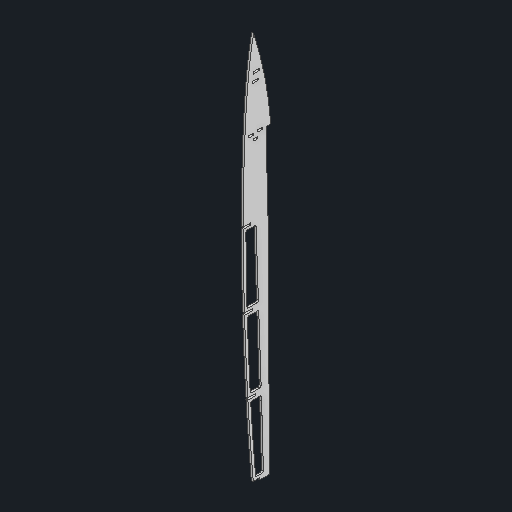
# Autodesk Inventor part: stringer
Saved by Autodesk Inventor 2024 (Build 280153000, 153)
## iProperties
Created: 2022-03-21
Part Number: stringer
Material: Generic
Document SubType Name: Modeling
Designer: kardo
Density: 1 g/cm^3
Appearance: Default
Mass: 41.3524 g
Surface Area: 339.584 cm^2
Volume: 41.3524 cm^3
Author: kardo
Autodesk Inventor part; units mm, degrees
ref_plane "YZ Plane" through (0, 0, 0) normal (1, 0, 0) x (0, 1, 0)
ref_plane "XZ Plane" through (0, 0, 0) normal (0, 1, 0) x (-1, 0, 0)
ref_plane "XY Plane" through (0, 0, 0) normal (0, 0, 1) x (1, 0, 0)
derived "parameters_frame.ipt"
derived "surface_body.ipt"
sketch "sk_long_outer" plane through (0, 0, 0) normal (1, 0, 0) x (0, 1, 0)
  line L0 (-345, 107.6209) -> (-345, -224.5198) construction
  line L1 (255, 107.6209) -> (255, -224.5198) construction
  line L2 (-465, 54.4) -> (375, 54.4) construction
  line L3 (-483, 0) -> (357, 0) construction
  line L4 (0, 107.6209) -> (0, -224.5198) construction
  line L5 (0, 14.144) -> (-345, 11.968)
  line L6 (-345, 11.968) -> (-345, 39.712)
  line L7 (-345, 39.712) -> (0, 54.4)
  line L8 (0, 54.4) -> (255, 36.448)
  line L9 (0, 0) -> (122.4, 9.6331)
  line L10 (122.4, 9.6331) -> (255, 36.448)
  line L11 (0, 14.144) -> (0, 0)
  line L12 (0, 14.144) -> (121.9006, 15.9783)
  line L13 (121.9006, 15.9783) -> (122.4, 9.6331)
sketch "sk_rail_sponson_tunnel" plane through (81.12, 0, 0) normal (1, 0, 0) x (0, 1, 0)
  line L0 (0, 0) -> (122.4, 9.6331)
  line L1 (111.1171, 152.996) -> (142.2856, -243.0375) construction
  spline S0 degree 2 poles (122.4, 9.6331) (190.08, 14.9596) (255, 36.448) knots 0 0 0 1 1 1
sketch "sk_rail_top_tunnel" plane through (81.12, 0, 0) normal (1, 0, 0) x (0, 1, 0)
  line L0 (255, 107.6209) -> (255, -224.5198) construction
  line L1 (0, 107.6209) -> (0, -224.5198) construction
  line L2 (-345, 107.6209) -> (-345, -224.5198) construction
  line L3 (-345, 0) -> (0, 0) construction
  line L4 (-172.5, 48.8998) -> (-172.5, 0) construction
  line L5 (0, 52.89) -> (37.026, 52.89) construction
  line L6 (37.026, 52.89) -> (80.784, 47.0555) construction
  line L7 (80.784, 47.0555) -> (112.2, 37.536) construction
  line L8 (112.2, 107.6209) -> (112.2, -224.5198) construction
  line L9 (0, 52.89) -> (255, 52.89) construction
  line L10 (-469.9275, 0) -> (379.2584, 0) construction
  spline S0 degree 3 poles (0, 52.89) (92.8353, 52.89) (195.0311, 49.5089) (255, 36.448) knots 0 0 0 0 1 1 1 1
  spline S1 degree 3 poles (0, 52.89) (37.026, 52.89) (80.784, 47.0555) (112.2, 37.536) knots 1 1 1 1 2 2 2 2
  spline S2 degree 4 poles (-345, 37.3935) (-258.8686, 45.1235) (-172.5923, 49.7074) (-86.3167, 52.89) (0, 52.89) knots 0 0 0 0 0 1 1 1 1 1
  point P0 (153, 48.7795)
  point P1 (112.2, 28.832)
  point P2 (-230.0001, 45.8224)
  point P3 (-114.9999, 50.9907)
sketch "sk_rail_bottom_tunnel" plane through (81.12, 0, 0) normal (1, 0, 0) x (0, 1, 0)
  line L0 (-241.5001, 19.2432) -> (11.22, 28.376)
  arc A0 (36.465, 28.832) -> (11.22, 28.376) centre (36.465, -670.197) ccw
  line L1 (36.465, 28.832) -> (112.2, 28.832)
  arc A1 (-262.2001, 18.586) -> (-241.5001, 19.2432) centre (-326.8578, 2381.2399) ccw
  line L2 (-345, 16.32) -> (-262.2001, 18.586)
  point P0 (0, 0)
ref_plane "plane_middle" through (0, 0, 0) normal (0, 1, 0) x (-1, 0, 0)
ref_plane "plane_tunnel_right" through (81.12, 0, 0) normal (1, 0, 0) x (0, 1, 0)
ref_plane "plane_tail_1" through (0, -114.9999, 0) normal (0, 1, 0) x (-1, 0, 0)
ref_plane "plane_tail_2" through (0, -230.0001, 0) normal (0, 1, 0) x (-1, 0, 0)
derived "stencil_frame.ipt"
sketch "sk_joint_locations" plane through (81.12, 0, 0) normal (1, 0, 0) x (0, 1, 0)
  line L0 (0, 0) -> (122.4, 9.6331) construction
  line L1 (36.465, 28.832) -> (112.2, 28.832) construction
  arc A0 (36.465, 28.832) -> (11.22, 28.376) centre (36.465, -670.197) ccw construction
  line L2 (-241.5001, 19.2432) -> (11.22, 28.376) construction
  line L3 (-345, 16.32) -> (-262.2001, 18.586) construction
  arc A1 (-262.2001, 18.586) -> (-241.5001, 19.2432) centre (-326.8578, 2381.2399) ccw construction
  line L4 (-122.4795, 3121.122) -> (270.8781, -1876.9598) construction
  line L5 (-230.0001, 3089.1136) -> (-230.0001, -1866.0023) construction
  line L6 (-114.9999, 3089.1136) -> (-114.9999, -1866.0023) construction
  line L7 (-345, 3089.1136) -> (-345, -1866.0023) construction
  line L8 (0, 3089.1136) -> (0, -1866.0023) construction
  line L9 (529.622, 47.2379) -> (-602.608, 2.7525) construction
  line L10 (-673.1615, -36.5999) -> (647.9226, 67.3717) construction
  line L11 (189.4528, 29.5173) -> (189.1111, 38.2146) construction
  line L12 (201.105, 36.5853) -> (201.7901, 27.8813) construction
  line L13 (0, 14.144) -> (121.9006, 15.9783) construction
  line L14 (-230.0001, 45.8224) -> (-230.0001, 19.6588) construction
  line L15 (-345, 37.3935) -> (-345, 16.32) construction
  line L16 (-114.9999, 50.9907) -> (-114.9999, 23.8147) construction
  line L17 (0, 52.89) -> (0, 27.9705) construction
  line L18 (119.1768, 50.5875) -> (119.7216, 43.6656) construction
  line L19 (120.2663, 36.7438) -> (119.7216, 43.6656) construction
  line L20 (120.2663, 36.7438) -> (120.8111, 29.822) construction
  line L21 (120.8111, 29.822) -> (121.3559, 22.9001) construction
  line L22 (121.3559, 22.9001) -> (121.9006, 15.9783) construction
  line L23 (0, 14.144) -> (0, 0) construction
  spline S0 degree 4 poles (-345, 37.3935) (-258.8686, 45.1235) (-172.5923, 49.7074) (-86.3167, 52.89) (0, 52.89) knots 0 0 0 0 0 1 1 1 1 1
  spline S1 degree 3 poles (0, 52.89) (92.8353, 52.89) (195.0311, 49.5089) (255, 36.448) knots 0 0 0 0 1 1 1 1
  spline S2 degree 2 poles (122.4, 9.6331) (190.08, 14.9596) (255, 36.448) knots 0 0 0 1 1 1
  line L24 (112.2, 37.536) -> (112.2, 28.832) construction
  line L25 (112.2, 35.848) -> (112.2, 30.52) construction
  point P0 (189.282, 33.8659)
  point P1 (201.4475, 32.2333)
  point P2 (-345, 26.8568)
  point P3 (-230.0001, 32.7406)
  point P4 (-114.9999, 37.4027)
  point P5 (0, 40.4303)
  point P6 (112.2, 33.184)
sketch "sk_stringer_base" plane through (81.12, 0, 0) normal (1, 0, 0) x (0, 1, 0)
  line L0 (0, 14.144) -> (-345, 11.968) construction
  spline S0 degree 4 poles (-345, 37.3935) (-258.8686, 45.1235) (-172.5923, 49.7074) (-86.3167, 52.89) (0, 52.89) knots 0 0 0 0 0 1 1 1 1 1 construction
  spline S1 degree 3 poles (0, 52.89) (37.026, 52.89) (80.784, 47.0555) (112.2, 37.536) knots 1 1 1 1 2 2 2 2 construction
  spline S2 degree 3 poles (0, 52.89) (92.8353, 52.89) (195.0311, 49.5089) (255, 36.448) knots 0 0 0 0 1 1 1 1 construction
  spline S3 degree 2 poles (122.4, 9.6331) (190.08, 14.9596) (255, 36.448) knots 0 0 0 1 1 1 construction
  line L1 (0, 0) -> (122.4, 9.6331) construction
  line L2 (-345, 16.32) -> (-262.2001, 18.586) construction
  arc A0 (-262.2001, 18.586) -> (-241.5001, 19.2432) centre (-326.8578, 2381.2399) ccw construction
  line L3 (-241.5001, 19.2432) -> (11.22, 28.376) construction
  arc A1 (36.465, 28.832) -> (11.22, 28.376) centre (36.465, -670.197) ccw construction
  line L4 (36.465, 28.832) -> (112.2, 28.832) construction
  line L5 (0, 2991.5273) -> (0, -1280.4843) construction
  line L6 (-345, 26.8568) -> (-345, 11.968)
  line L7 (-345, 11.968) -> (0, 14.144)
  line L8 (119.3465, 10.1952) -> (118.832, 16.7322)
  line L9 (0, 14.144) -> (0, 14.944)
  line L10 (0, 14.944) -> (118.832, 16.7322)
  line L11 (-345, 26.8568) -> (-342, 26.8568)
  line L12 (-342, 26.8568) -> (-342, 36.8582)
  line L13 (-230.0001, 32.7406) -> (-227.0001, 32.7406)
  line L14 (-227.0001, 32.7406) -> (-227.0001, 45.1951)
  line L15 (-230.0001, 32.7406) -> (-230.0001, 45.0211)
  line L16 (-114.9999, 37.4027) -> (-114.9999, 50.1903)
  line L17 (-114.9999, 37.4027) -> (-111.9999, 37.4027)
  line L18 (-111.9999, 37.4027) -> (-111.9999, 50.2837)
  line L19 (0, 52.09) -> (0, 40.4303)
  line L20 (0, 40.4303) -> (3, 40.4303)
  line L21 (3, 40.4303) -> (3, 52.0888)
  line L22 (119.7216, 43.6656) -> (120.2663, 36.7438)
  line L23 (120.2663, 36.7438) -> (117.2756, 36.5084)
  line L24 (117.2756, 36.5084) -> (116.7308, 43.4303)
  line L25 (116.7308, 43.4303) -> (119.7216, 43.6656)
  line L26 (120.8111, 29.822) -> (117.8203, 29.5866)
  line L27 (117.8203, 29.5866) -> (118.3651, 22.6647)
  line L28 (118.3651, 22.6647) -> (121.3559, 22.9001)
  line L29 (120.8111, 29.822) -> (121.3559, 22.9001)
  line L30 (189.1111, 38.2146) -> (189.4528, 29.5173)
  line L31 (201.105, 36.5853) -> (201.7901, 27.8813)
  line L32 (201.7901, 27.8813) -> (198.7993, 27.646)
  line L33 (198.7993, 27.646) -> (198.1143, 36.35)
  line L34 (198.1143, 36.35) -> (201.105, 36.5853)
  line L35 (189.1111, 38.2146) -> (186.1134, 38.0968)
  line L36 (186.1134, 38.0968) -> (186.4551, 29.3995)
  line L37 (186.4551, 29.3995) -> (189.4528, 29.5173)
  line L38 (122.3372, 10.4306) -> (119.3465, 10.1952)
  line L39 (109.2, 35.848) -> (112.2, 35.848)
  line L40 (112.2, 35.848) -> (112.2, 30.52)
  line L41 (112.2, 30.52) -> (109.2, 30.52)
  line L42 (109.2, 30.52) -> (109.2, 35.848)
  spline S4 degree 5 poles (-342, 36.8582) (-273.7802, 42.9173) (-205.3987, 47.149) (-136.9758, 50.2102) (-68.4884, 52.0902) (0, 52.09) knots 0 0 0 0 0 0 1 1 1 1 1 1
  spline S5 degree 5 poles (0, 52.09) (14.1126, 52.09) (28.2252, 52.0249) (42.3374, 51.8877) (70.3021, 51.4557) (98.2587, 50.655) (112.105, 50.1551) (138.5853, 48.9703) (165.0353, 47.2425) (177.6496, 46.2711) (200.7384, 44.1675) (223.7378, 41.2476) (234.1569, 39.7078) (244.5404, 37.9065) (254.8298, 35.6663) knots 0 0 0 0 0 0 0.275917 0.275917 0.275917 0.546795 0.546795 0.546795 0.794123 0.794123 0.794123 1 1 1 1 1 1
  spline S6 degree 4 poles (254.7486, 37.2075) (222.6091, 26.5695) (189.6306, 18.4466) (156.0872, 13.0866) (122.3372, 10.4306) knots 0 0 0 0 0 1 1 1 1 1
  point P0 (251.9318, 36.2831)
  point P1 (121.9006, 15.9783)
  dimension "d4" = 0.8
  dimension "d14" = 0.8
  dimension "d8" = 0.8
  dimension "d9" = 3
  dimension "d11" = 3
  dimension "d16" = 3
  dimension "d17" = 0.8
  constraints: 74 end point, 12 perpendicular, 7 vertical, 6 equal length, 6 parallel, 2 coincident, 2 collinear, 2 horizontal, 18 other
  measures "d8" distance of L7.end L9.end
  measures "d9" distance of L6.start L11.end
  measures "d11" distance of L19.end L20.end
  measures "d16" distance between parallel lines of L40 L42
  measures "d17" distance from line of point (121.901, 15.978) L10
extrude "thicken" add sketch "sk_stringer_base" along normal blind 3 contours L11 L12 S4 L15 L13 L14 L16 L17 L18 L19 L20 L21 S5 S6 L38 L8 L10 L9 L7 L6
sketch "sk_cut_weight" plane through (81.12, 0, 0) normal (1, 0, 0) x (0, 1, 0)
  spline S0 degree 4 poles (-345, 37.3935) (-258.8686, 45.1235) (-172.5923, 49.7074) (-86.3167, 52.89) (0, 52.89) knots 0 0 0 0 0 1 1 1 1 1 construction
  spline S1 degree 3 poles (0, 52.89) (37.026, 52.89) (80.784, 47.0555) (112.2, 37.536) knots 1 1 1 1 2 2 2 2 construction
  line L0 (36.465, 28.832) -> (112.2, 28.832) construction
  arc A0 (36.465, 28.832) -> (11.22, 28.376) centre (36.465, -670.197) ccw construction
  line L1 (-241.5001, 19.2432) -> (11.22, 28.376) construction
  arc A1 (-262.2001, 18.586) -> (-241.5001, 19.2432) centre (-326.8578, 2381.2399) ccw construction
  line L2 (-345, 16.32) -> (-262.2001, 18.586) construction
  line L3 (112.2, 37.536) -> (112.2, 28.832) construction
  line L4 (108.4873, 33.632) -> (36.465, 33.632)
  arc A2 (36.465, 33.632) -> (11.0467, 33.1729) centre (36.465, -670.197) ccw
  line L5 (11.0467, 33.1729) -> (-241.6735, 24.0401)
  arc A3 (-262.3314, 23.3842) -> (-241.6735, 24.0401) centre (-326.8578, 2381.2399) ccw
  line L6 (-262.3314, 23.3842) -> (-338, 21.3134)
  line L7 (-345, 16.32) -> (-345, 37.3935) construction
  line L8 (-342, 46.2922) -> (-342, 7.6751) construction
  line L9 (-227.0001, 59.5201) -> (-227.0001, 2.898) construction
  line L10 (-111.9999, 68.9991) -> (-111.9999, 15.2181) construction
  line L11 (0, 2991.5273) -> (0, -1280.4843) construction
  line L12 (-230.0001, 2991.5273) -> (-230.0001, -1280.4843) construction
  line L13 (-114.9999, 2991.5273) -> (-114.9999, -1280.4843) construction
  line L14 (-338, 21.3134) -> (-338, 33.1956)
  line L15 (-234.0001, 40.7786) -> (-234.0001, 24.3174)
  line L16 (-223.0001, 41.4174) -> (-223.0001, 24.7149)
  line L17 (-118.9999, 46.0602) -> (-118.9999, 28.4733)
  line L18 (-107.9999, 46.4032) -> (-107.9999, 28.8708)
  line L19 (-4, 48.0874) -> (-4, 32.6291)
  spline S2 degree 5 poles (-338, 33.1956) (-270.5733, 39.1068) (-202.9921, 43.2515) (-135.37, 46.2518) (-67.6854, 48.0902) (0, 48.09) knots 0 0 0 0 0 0 1 1 1 1 1 1
  spline S3 degree 5 poles (0, 48.09) (7.6357, 48.0899) (15.2714, 47.8806) (22.8997, 47.4965) (38.2518, 46.3949) (53.5443, 44.6516) (61.2292, 43.6141) (75.3782, 41.394) (89.4128, 38.543) (95.8175, 37.089) (102.1841, 35.4696) (108.4873, 33.632) knots 0 0 0 0 0 0 0.347809 0.347809 0.347809 0.700936 0.700936 0.700936 1 1 1 1 1 1
  point P0 (0, 0)
  dimension "d20" = 4.8
  dimension "d21" = 3
  dimension "d22" = 3
  dimension "d23" = 3
  dimension "d25" = 4
  dimension "d26" = 4
  dimension "d27" = 4
  dimension "d28" = 4
  dimension "d29" = 4
  dimension "d30" = 4
  constraints: 29 end point, 10 parallel, 5 point on line, 4 point on circle, 2 centre point, 16 other
  measures "d21" distance between parallel lines of L7 L8
  measures "d22" distance between parallel lines of L12 L9
  measures "d23" distance between parallel lines of L13 L10
  measures "d25" distance between parallel lines of L8 L14
  measures "d26" distance between parallel lines of L12 L15
  measures "d27" distance between parallel lines of L9 L16
  measures "d28" distance between parallel lines of L17 L13
  measures "d29" distance between parallel lines of L18 L10
  measures "d30" distance between parallel lines of L19 L11
extrude "cut_weight" cut sketch "sk_cut_weight" along normal through all both and the other way through all contours L19 L5 L18 S2 | L17 L5 L16 S2 | L15 L5 A3 L6 L14 S2
fillet "rounding" radius 2 12 edges at (82.62, -4, 32.6291) (82.62, -4, 48.0874) (82.62, -118.9999, 46.0602) (82.62, -234.0001, 40.7786) (82.62, -234.0001, 24.3174) (82.62, -118.9999, 28.4733) (82.62, -338, 21.3134) (82.62, -223.0001, 24.7149) (82.62, -107.9999, 28.8708) (82.62, -107.9999, 46.4032) (82.62, -223.0001, 41.4174) (82.62, -338, 33.1956)
equation "\"d4\" = shell_thickness"
equation "\"d14\" = shell_thickness"
equation "\"d8\" = shell_thickness"
equation "\"d9\" = bulkhead_thickness"
equation "\"d11\" = bulkhead_thickness"
equation "\"d16\" = bulkhead_thickness"
equation "\"d17\" = shell_thickness"
equation "\"d12\" = stringer_thickness"
equation "\"d20\" = bulkhead_inset + shell_thickness"
equation "\"d21\" = bulkhead_thickness"
equation "\"d22\" = bulkhead_thickness"
equation "\"d23\" = bulkhead_thickness"
equation "\"d25\" = bulkhead_inset"
equation "\"d26\" = bulkhead_inset"
equation "\"d27\" = bulkhead_inset"
equation "\"d28\" = bulkhead_inset"
equation "\"d29\" = bulkhead_inset"
equation "\"d30\" = bulkhead_inset"
equation "\"d34\" = 0.5 * bulkhead_inset"
equation "\"shell_thickness\" = 0.8"
equation "\"bulkhead_thickness\" = 3"
equation "\"stringer_thickness\" = 3"
equation "\"bulkhead_inset\" = 4"
body "Solid1"
